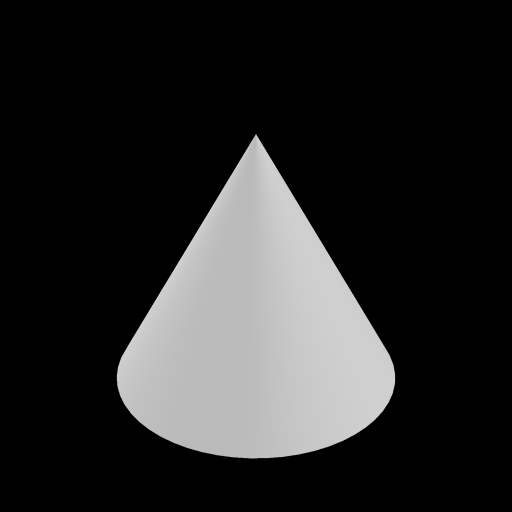
# Autodesk Inventor part: CoolerFunnel
Saved by Autodesk Inventor 2023 (Build 270158000, 158)
## iProperties
Created: 2023-09-14
Part Number: CoolerFunnel
Material: Generic
Document SubType Name: Modeling
Designer: tandu
Density: 1 g/cm^3
Appearance: Default
Author: tandu
Autodesk Inventor part; units mm, degrees
ref_plane "YZ Plane" through (0, 0, 0) normal (1, 0, 0) x (0, 1, 0)
ref_plane "XZ Plane" through (0, 0, 0) normal (0, 1, 0) x (-1, 0, 0)
ref_plane "XY Plane" through (0, 0, 0) normal (0, 0, 1) x (1, 0, 0)
sketch "Sketch1" plane through (0, 0, 0) normal (0, 0, 1) x (1, 0, 0)
  line L0 (-28.575, 0) -> (28.575, 0)
  line L1 (0, 0) -> (25.4, 0)
  line L2 (25.4, 0) -> (25.4, 7.62)
  line L3 (0, 0) -> (0, 62.0905)
  line L4 (0, 62.0905) -> (25.4, 7.62)
  line L5 (25.4, 7.62) -> (0, 7.62)
  dimension "d0" = 57.15
  dimension "d1" = 3.175
  dimension "d2" = 7.62
  dimension "d3" = 65
  constraints: 12 end point, 2 point on line, 2 vertical, 1 coincident, 1 horizontal, 1 midpoint, 1 perpendicular
  measures "d0" distance of L0.start L0.end
  measures "d1" distance of L0.end L1.end
  measures "d2" distance of L1.end L2.end
  measures "d3" angle of L0 L4
revolve "Revolution1" add sketch "Sketch1" angle 360 about axis through (0, 0, 0) along (0, 1, 0) contours L3 L4 L5
sketch "Sketch3" plane through (0, 7.62, 0) normal (0, -1, 0) x (1, 0, 0)
  line L0 (7.479, 0) -> (3.7395, -6.477)
  line L1 (3.7395, -6.477) -> (-3.7395, -6.477)
  line L2 (-3.7395, -6.477) -> (-7.479, 0)
  line L3 (-7.479, 0) -> (-3.7395, 6.477)
  line L4 (-3.7395, 6.477) -> (3.7395, 6.477)
  line L5 (3.7395, 6.477) -> (7.479, 0)
  point P0 (0, 0)
  point P1 (0, 0)
  dimension "d8" = 12.954
  constraints: 12 end point, 1 coincident, 1 horizontal, 13 other
  measures "d8" distance of L0.end L4.end
extrude "HexSlot" cut sketch "Sketch3" against normal blind 6.35
sketch "Sketch2" plane through (-3.6662, 0, 6.35) normal (0, -1, 0) x (1, 0, 0)
  line L0 (10.9985, -6.35) -> (7.3323, 0) projected
  line L1 (7.3323, 0) -> (0, 0) projected
  line L2 (0, 0) -> (-3.6662, -6.35) projected
  line L3 (-3.6662, -6.35) -> (0, -12.7) projected
  line L4 (0, -12.7) -> (7.3323, -12.7) projected
  line L5 (7.3323, -12.7) -> (10.9985, -6.35) projected
  circle A0 centre (3.6662, -6.35) radius 26.035 projected
  arc A1 (17.5648, 13.044) -> (13.5125, 15.3836) centre (3.6662, -6.35) ccw projected
  circle A2 centre (3.6662, -6.35) radius 23.86
  point P0 (13.5125, 15.3836)
  constraints: 1 coincident, 3 other
body "Solid1"
